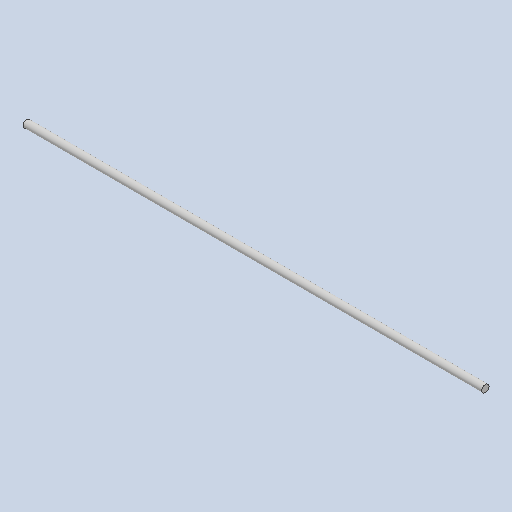
# Autodesk Inventor part: rod
Saved by Autodesk Inventor 2023 (Build 270158000, 158)
## iProperties
Created: 2022-08-28
Part Number: rod
Material: Generic
Document SubType Name: Modeling
Designer: Nathann
Density: 1 g/cm^3
Appearance: Default
Author: Nathann
Autodesk Inventor part; units mm, degrees
ref_plane "YZ Plane" through (0, 0, 0) normal (1, 0, 0) x (0, 1, 0)
ref_plane "XZ Plane" through (0, 0, 0) normal (0, 1, 0) x (-1, 0, 0)
ref_plane "XY Plane" through (0, 0, 0) normal (0, 0, 1) x (1, 0, 0)
sketch "Sketch1" plane through (0, 0, 0) normal (1, 0, 0) x (0, 1, 0)
  circle A0 centre (0, 0) radius 4
  dimension "d0" = 8
  constraints: 1 centre point, 1 coincident
  measures "d0" diameter of A0
extrude "Extrusion1" add sketch "Sketch1" along normal blind 500
equation "\"d0\" = RodDiameter"
equation "\"d1\" = RodLenght"
equation "\"RodDiameter\" = 8"
equation "\"VerticalBearingOD\" = 16"
equation "\"PrintingClearance\" = 0.2"
equation "\"TubeID\" = 18"
equation "\"XLinearBearingOD\" = 19"
equation "\"RodLenght\" = 500"
body "Solid1"
